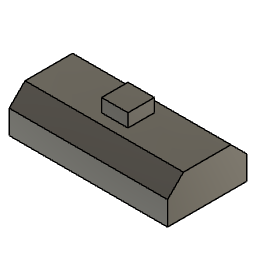
Projet Fabnum V2 v1 (Autodesk Fusion 360 design; units mm, degrees)
Autodesk Fusion 360 part; units mm, degrees
sketch "Esquisse1" plane through (0, 0, 0) normal (0, 0, 1) x (1, 0, 0)
  line L0 (0, 0) -> (300, 0)
  line L1 (300, 0) -> (300, 150)
  line L2 (300, 150) -> (0, 150)
  line L3 (0, 150) -> (0, 0)
  constraint horizontal L0
  constraint vertical L1
  constraint horizontal L2
  constraint vertical L3
  constraint coincident L0.start L3.end
extrude "Extrusion1" add sketch "Esquisse1" along normal blind 75
chamfer "Chanfrein1" distance 30 angle 45 1 edges at (150, 0, 75)
chamfer "Chanfrein2" distance 30 angle 45 1 edges at (150, 150, 75)
box "BoitePrimitive1" add length 50 width 50 height 25 placed x (0, -1, 0) y (1, 0, 0) z (0, 0, 1) at (125, 100, 75)
